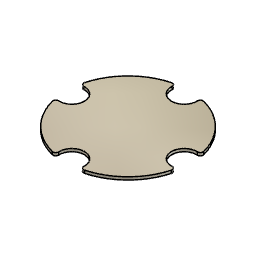
silver contact part v4 (Autodesk Fusion 360 design; units mm, degrees)
Autodesk Fusion 360 part; units mm, degrees
sketch "Sketch1" plane through (0, 0, 0) normal (0, 1, 0) x (1, 0, 0)
  circle A0 centre (0, 0) radius 10 construction
  circle A1 centre (10, 0) radius 2.25
  circle A2 centre (0, 10) radius 2.25
  circle A3 centre (-10, 0) radius 2.25
  circle A4 centre (0, -10) radius 2.25
  circle A5 centre (0, 0) radius 11
  dimension "d1" = 20
  dimension "d2" = 4.5
  dimension "d4" = 360
  dimension "d5" = 22
  constraint coincident A0.centre A5.centre
  constraint coincident A0 A1.centre
  constraint horizontal A0.centre A1.centre
  constraint concentric A0 A5
  measures "d1" diameter of A0
  measures "d2" diameter of A1
  measures "d5" diameter of A5
extrude "Extrude1" add sketch "Sketch1" along normal blind 0.5 contours A1 A2 A3 A4 A5
fillet "Fillet1" radius 0.5 8 edges at (-2.1042, 0.25, 10.7969) (2.1042, 0.25, 10.7969) (-10.7969, 0.25, 2.1042) (-10.7969, 0.25, -2.1042) (-2.1042, 0.25, -10.7969) (2.1042, 0.25, -10.7969) (10.7969, 0.25, -2.1042) (10.7969, 0.25, 2.1042)
